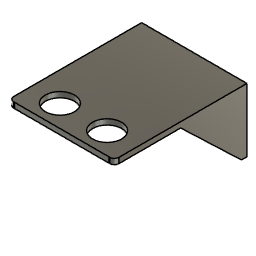
hcsr04_support_v4 (Autodesk Fusion 360 design; units mm, degrees)
Autodesk Fusion 360 part; units mm, degrees
sketch "Esboço1" plane through (0, 0, 0) normal (0, 0, 1) x (1, 0, 0)
  line L0 (0, 0) -> (52, 0)
  line L1 (0, -70) -> (0, 0)
  line L2 (52, -35) -> (0, -35) construction
  circle A0 centre (13, -58) radius 8
  line L3 (13, -70) -> (13, -66) construction
  line L4 (0, -58) -> (5, -58) construction
  line L5 (21, -58) -> (31, -58) construction
  circle A1 centre (39, -58) radius 8
  line L6 (39, -66) -> (39, -70) construction
  line L7 (47, -58) -> (52, -58) construction
  line L8 (0, -70) -> (52, -70)
  line L9 (52, -70) -> (52, 0)
  line L10 (26, -70) -> (26, 0) construction
  line L11 (11, -27.5) -> (41, -27.5)
  line L12 (41, -27.5) -> (41, -42.5)
  line L13 (41, -42.5) -> (11, -42.5)
  line L14 (11, -42.5) -> (11, -27.5)
  line L15 (11, -27.5) -> (41, -42.5) construction
  line L16 (41, -27.5) -> (11, -42.5) construction
  line L17 (52, -70) -> (55, -70)
  line L18 (0, -70) -> (-3, -70)
  line L19 (55, -70) -> (55, 0)
  line L20 (55, 0) -> (52, 0)
  line L21 (-3, -70) -> (-3, 0)
  line L22 (-3, 0) -> (0, 0)
  point P0 (26, -35)
  dimension "d1" = 70
  dimension "d5" = 8
  dimension "d7" = 4
  dimension "d8" = 5
  dimension "d9" = 10
  dimension "d10" = 16
  dimension "d11" = 4
  dimension "d12" = 5
  dimension "d14" = 52
  dimension "d15" = 30
  dimension "d16" = 15
  dimension "d32" = 3
  dimension "d33" = 3
  constraint horizontal L0
  constraint vertical L1
  constraint coincident L0.start L1.end
  constraint midpoint L1 L2.end
  constraint coincident A0 L3.end
  constraint coincident L1 L4.start
  constraint coincident A0 L4.end
  constraint perpendicular L1 L4
  constraint coincident A0 L5.start
  constraint coincident L5.end A1
  constraint coincident A1 L6.start
  constraint coincident A1 L7.start
  constraint horizontal L7
  constraint perpendicular L1 L8
  constraint perpendicular L0 L9
  constraint coincident L9 L2.start
  constraint midpoint L8 L10.start
  constraint midpoint L0 L10.end
  constraint horizontal L11
  constraint perpendicular L11 L12
  constraint parallel L11 L13
  constraint parallel L12 L14
  constraint coincident L15 P0
  constraint coincident L16 P0
  constraint midpoint L10 P0
  constraint perpendicular L9 L17
  constraint perpendicular L1 L18
  constraint perpendicular L17 L19
  constraint perpendicular L9 L20
  constraint perpendicular L18 L21
  constraint perpendicular L1 L22
  measures "d1" distance of L0.start L1.start
  measures "d5" radius of A0
  measures "d7" distance of L3.start L3.end
  measures "d8" distance of L4.start L4.end
  measures "d9" distance of L5.start L5.end
  measures "d10" diameter of A1
  measures "d11" distance of L6.end L6.start
  measures "d12" distance of L7.start L7.end
  measures "d14" distance of L1.start L8.end
  measures "d15" distance of L12.end L13.end
  measures "d16" distance of L11.end L12.end
  measures "d32" distance of L8.end L17.end
  measures "d33" distance of L1.start L18.end
extrude "Extrusão1" add sketch "Esboço1" along normal blind 3 contours L0 L1 L8 L9 | L1 L18 L21 L22 | L9 L17 L19 L20 | L11 L12 L13 L14
ref_plane "Plano de trabalho1" through (26, 0, 1.5) normal (0, 1, 0) x (-1, 0, 0)
sketch "Esboço2" plane through (0, 0, 0) normal (0, 1, 0) x (1, 0, 0)
  line L0 (0, 0) -> (0, 32)
  line L1 (0, 32) -> (52, 32)
  line L2 (52, 32) -> (52, 0)
  line L3 (26, 0) -> (26, 32) construction
  line L4 (52, 16) -> (0, 16) construction
  circle A0 centre (26, 16) radius 8
  circle A1 centre (47.5, 4.5) radius 1.5
  circle A2 centre (4.5, 4.5) radius 1.5
  circle A3 centre (47.5, 27.5) radius 1.5
  line L5 (49, 32) -> (49, 29) construction
  line L6 (52, 29) -> (47.5, 29) construction
  line L7 (49, 29) -> (49, 27.5) construction
  circle A4 centre (4.5, 27.5) radius 1.5
  line L8 (3, 32) -> (3, 29) construction
  line L9 (0, 29) -> (4.5, 29) construction
  line L10 (3, 29) -> (3, 27.5) construction
  line L11 (52, 0) -> (52, -3)
  line L12 (52, -3) -> (0, -3)
  line L13 (0, 0) -> (0, -3)
  line L14 (0, -3) -> (-3, -3)
  line L15 (-3, -3) -> (-3, 32)
  line L16 (-3, 32) -> (0, 32)
  dimension "d22" = 16
  dimension "d26" = 1.5
  dimension "d34" = 3
  constraint vertical L0
  constraint horizontal L1
  constraint vertical L2
  constraint midpoint L1 L3.end
  constraint midpoint L2 L4.start
  constraint midpoint L0 L4.end
  constraint midpoint L3 A0.centre
  constraint symmetric L3 A1 A2
  constraint symmetric L4 A1 A3
  constraint symmetric L4 A2 A4
  constraint coincident L0.start L13.start
  constraint perpendicular L12 L13
  constraint perpendicular L13 L14
  constraint perpendicular L14 L15
  constraint perpendicular L0 L16
  measures "d22" diameter of A0
  measures "d26" radius of A1
  measures "d34" distance of L12.end L14.end
extrude "Extrusão2" add sketch "Esboço2" along normal blind 3
ref_plane "Plano de trabalho2" through (52, 1.5, -14.5) normal (1, 0, 0) x (0, 0, -1)
sketch "Esboço3" plane through (52, 0, 0) normal (1, 0, 0) x (0, 1, 0)
  line L0 (3, -32) -> (0, -32)
  line L1 (-33.5, 0) -> (0, 0)
  line L2 (-33.5, 0) -> (0, -32)
  line L3 (0, -32) -> (3, -32)
  line L4 (3, -32) -> (3, 0)
  line L5 (0, 0) -> (0, 3)
  line L6 (0, 3) -> (3, 3)
  line L7 (3, 3) -> (3, 0)
  constraint horizontal L0
  constraint horizontal L1
  constraint perpendicular L1 L4
  constraint coincident L1.end L5.start
  constraint perpendicular L1 L5
  constraint perpendicular L4 L6
  constraint perpendicular L1 L7
  constraint coincident L5 L1.end
extrude "Extrusão3" add sketch "Esboço3" along normal blind 3
ref_plane "Plano de trabalho3" through (-3, -33.5, -14.5) normal (-1, 0, 0) x (0, -1, 0)
sketch "Esboço4" plane through (-3, 0, 0) normal (-1, 0, 0) x (0, -1, 0)
  line L0 (0, 0) -> (69, 0)
  line L1 (33, 0) -> (0, -32)
  line L2 (0, -32) -> (0, 0)
  constraint horizontal L0
  constraint coincident L0.start L2.end
  constraint perpendicular L0 L2
  constraint coincident L2 L0.start
  constraint coincident L0 L1.start
extrude "Extrusão4" add sketch "Esboço4" against normal blind 3
fillet "Arredondamento1" radius 2.5 1 edges at (-3, -70, 1.5)
fillet "Arredondamento2" radius 2.5 1 edges at (55, -70, 1.5)
